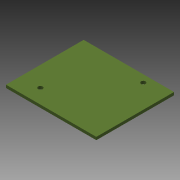
# Autodesk Inventor part: SMD_Platine
Saved by Autodesk Inventor 2015 (Build 190159000, 159)
## iProperties
Created: 2015-03-02
Part Number: SMD_Platine
Material: Generisch
Document SubType Name: Modeling
Designer: TowerSebi
Density: 1 g/cm^3
Appearance: Olivgrün
Author: TowerSebi
Autodesk Inventor part; units mm, degrees
ref_plane "YZ Plane" through (0, 0, 0) normal (1, 0, 0) x (0, 1, 0)
ref_plane "XZ Plane" through (0, 0, 0) normal (0, 1, 0) x (-1, 0, 0)
ref_plane "XY Plane" through (0, 0, 0) normal (0, 0, 1) x (1, 0, 0)
sketch "Skizze1" plane through (0, 0, 0) normal (0, 0, 1) x (1, 0, 0)
  line L0 (0, 0) -> (63.5, 0)
  line L1 (63.5, 0) -> (63.5, 54.6)
  line L2 (63.5, 54.6) -> (0, 54.6)
  line L3 (0, 54.6) -> (0, 0)
  circle A0 centre (14, 10.2) radius 1.6
  circle A1 centre (47, 49.5) radius 1.6
  dimension "d0" = 54.6
  dimension "d1" = 63.5
  dimension "d2" = 3.2
  dimension "d3" = 3.2
  dimension "d4" = 14
  dimension "d5" = 10.2
  dimension "d6" = 49.5
  dimension "d7" = 47
  dimension "d10" = 33
  dimension "d11" = 39.3
  constraints: 8 end point, 2 centre point, 2 parallel, 1 horizontal, 1 perpendicular
  measures "d0" distance of L2.end L0.start
  measures "d1" distance of L0.start L0.end
  measures "d2" diameter of A0
  measures "d3" diameter of A1
  measures "d4" distance from line of L3 A0.centre
  measures "d5" distance from line of L0 A0.centre
  measures "d6" distance from line of L0 A1.centre
  measures "d7" distance from line of L3 A1.centre
  measures "d10" horizontal distance of A1.centre A0.centre
  measures "d11" vertical distance of A0.centre A1.centre
extrude "Extrusion1" add sketch "Skizze1" along normal blind 2
